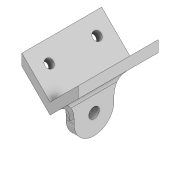
# Autodesk Inventor part: soporte_medio
Saved by Autodesk Inventor 2022 (Build 260153000, 153)
## iProperties
Created: 2022-11-01
Part Number: soporte_medio
Material: Genérico
Document SubType Name: Modeling
Designer: Jorge
Density: 1 g/cm^3
Appearance: Valor por defecto
Author: Jorge
Autodesk Inventor part; units mm, degrees
ref_plane "YZ Plane" through (0, 0, 0) normal (1, 0, 0) x (0, 1, 0)
sketch "Boceto1" plane through (0, 0, 0) normal (0, 0, 1) x (1, 0, 0)
  line L0 (0, 0) -> (10.6066, 10.6066)
  line L1 (0, 0) -> (-10.6066, 10.6066)
  line L2 (-10.6066, 10.6066) -> (-10.6066, 6.364)
  line L3 (-10.6066, 6.364) -> (0, -4.2426)
  line L4 (0, -4.2426) -> (10.6066, 6.364)
  line L5 (10.6066, 6.364) -> (10.6066, 10.6066)
  dimension "d0" = 15
  dimension "d2" = 15
  dimension "d6" = 3
  dimension "d7" = 3
  constraints: 12 end point, 2 vertical, 1 perpendicular
  measures "d0" distance of L0.start L0.end
  measures "d2" distance of L0.start L1.end
  measures "d6" distance between parallel lines of L3 L1
  measures "d7" distance between parallel lines of L0 L4
extrude "Extrusión1" add sketch "Boceto1" along normal blind 30
ref_plane "Plano de trabajo1" through (0, 0, 15) normal (0, 0, 1) x (1, 0, 0)
sketch "Boceto2" plane through (0, 0, 15) normal (0, 0, 1) x (1, 0, 0)
  line L0 (-10.6066, 6.364) -> (0, -4.2426) construction
  line L1 (0, -4.2426) -> (10.6066, 6.364) construction
  line L2 (10.6066, 6.364) -> (10.6066, 10.6066) construction
  line L3 (10.6066, 10.6066) -> (0, 0) construction
  line L4 (0, 0) -> (-10.6066, 10.6066) construction
  line L5 (-10.6066, 10.6066) -> (-10.6066, 6.364) construction
  line L6 (-10.6066, 6.364) -> (0, -4.2426) projected
  line L7 (-1.5, -2.7426) -> (-1.5, -17.7426)
  line L8 (1.5, -2.7426) -> (1.5, -17.7426)
  line L9 (-1.5, -17.7426) -> (1.5, -17.7426)
  line L10 (0, -4.2426) -> (10.6066, 6.364) projected
  line L11 (0, -4.2426) -> (1.5, -2.7426)
  line L12 (-1.5, -2.7426) -> (0, -4.2426)
  dimension "d10" = 3
  dimension "d11" = 1.5
  dimension "d12" = 15
  constraints: 10 end point, 5 point on line, 2 vertical, 1 horizontal
  measures "d10" distance of L7.end L8.end
  measures "d11" distance from line of L0.end L7
  measures "d12" distance of L7.start L7.end
extrude "Extrusión2" add sketch "Boceto2" along normal mid plane 15
fillet "Empalme1" radius 7.5 2 edges at (0, -17.7426, 22.5) (0, -17.7426, 7.5)
fillet "Empalme2" radius 4 6 edges at (0.75, -3.4926, 22.5) (-0.75, -3.4926, 22.5) (-0.75, -3.4926, 7.5) (0.75, -3.4926, 7.5) (-1.5, -2.7426, 15) (1.5, -2.7426, 15)
sketch "Boceto3" plane through (1.5, -10.2426, 15) normal (1, 0, 0) x (0, 0, -1)
  line L0 (-8.6716, 5.8431) -> (8.6716, 5.8431) construction
  ellipse E0 centre (-11.5, 1.8431) end of major axis (-11.5, 7.5) minor radius 4 (-7.5, 1.8431) -> (-8.6716, 5.8431) ccw construction
  line L1 (-7.5, 0) -> (-7.5, 1.8431) construction
  arc A0 (-7.5, 0) -> (7.5, 0) centre (0, 0) ccw construction
  line L2 (7.5, 1.8431) -> (7.5, 0) construction
  ellipse E1 centre (11.5, 1.8431) end of major axis (11.5, 7.5) minor radius 4 (8.6716, 5.8431) -> (7.5, 1.8431) ccw construction
  circle A1 centre (0, 0) radius 2
  point P0 (15, 10.2426)
  dimension "d17" = 4
  constraints: 1 centre point, 1 coincident, 2 other
  measures "d17" diameter of A1
extrude "Extrusión3" cut sketch "Boceto3" against normal through all
sketch "Boceto4" plane through (10.6066, 6.364, 30) normal (0.7071068, -0.7071068, 0) x (-0.7071068, -0.7071068, 0)
  line L0 (15, 26.5) -> (11.2218, 26.5) construction
  line L1 (15, 30) -> (15, 26.5) construction
  line L2 (15, 30) -> (0, 30) construction
  line L3 (0, 30) -> (0, 0) construction
  line L4 (15, 0) -> (0, 0) construction
  line L5 (15, 3.5) -> (15, 0) construction
  line L6 (11.2218, 3.5) -> (15, 3.5) construction
  line L7 (11.2218, 26.5) -> (11.2218, 3.5) construction
  line L8 (-3, 0) -> (12, 0) construction
  line L9 (3, 0) -> (3, 30) construction
  line L10 (0, 30) -> (0, 0) construction
  line L11 (0, 6) -> (11.2218, 6) construction
  line L12 (0, 24) -> (11.2218, 24) construction
  line L13 (11.2218, 26.5) -> (11.2218, 3.5) construction
  line L14 (11.2218, 15) -> (0, 15) construction
  circle A0 centre (3, 6) radius 1.6
  circle A1 centre (3, 24) radius 1.6
  point P0 (12, 30)
  dimension "d20" = 3.2
  dimension "d21" = 3.2
  dimension "d22" = 18
  dimension "d23" = 9
  dimension "d24" = 3
  constraints: 10 point on line, 8 end point, 2 centre point, 2 midpoint, 2 perpendicular, 1 parallel
  measures "d20" diameter of A0
  measures "d21" diameter of A1
  measures "d22" distance between parallel lines of L12 L11
  measures "d23" distance between parallel lines of L14 L11
  measures "d24" distance between parallel lines of L3 L9
extrude "Extrusión4" cut sketch "Boceto4" against normal through all
ref_plane "Plano de trabajo2" through (0, -10.2426, 15) normal (1, 0, 0) x (0, 0, -1)
mirror "Simetría1" about plane through (0, -10.2426, 15) normal (1, 0, 0) of "Extrusión4"
equation "\"d11\" = 0.5 * d10"
equation "\"d23\" = 0.5 * d22"
